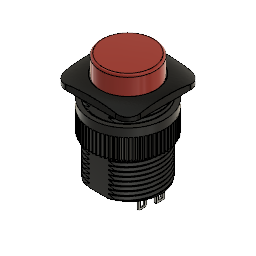
LED Pushbutton (Autodesk Fusion 360 design; units mm, degrees)
Autodesk Fusion 360 part; units mm, degrees
note: some values were not read from the file. Chosen so that the rebuilt part matches the saved one: which face or edge a step refers to. Set by a fixed rule: which sketch regions a step uses.
sketch "Sketch1" plane through (0, 0, 0) normal (0, 0, 1) x (1, 0, 0) in component "Top"
  circle A0 centre (0, 0) radius 6.5
  dimension "d1" = 13
  constraint coincident A0.centre origin
  measures "d1" diameter of A0
extrude "Extrude1" add sketch "Sketch1" along normal blind 6.3 makes body 1 in component "Top"
sketch "Sketch1 (2)" plane through (0, 0, 0) normal (0, 0, 1) x (1, 0, 0) in component "Bezel"
  line L0 (9, 9) -> (-9, 9)
  line L1 (-9, 9) -> (-9, -9)
  line L2 (-9, -9) -> (9, -9)
  line L3 (9, -9) -> (9, 9)
  line L4 (9, 9) -> (-9, -9) construction
  line L5 (-9, 9) -> (9, -9) construction
  dimension "d4" = 18
  dimension "d5" = 18
  constraint horizontal L0
  constraint perpendicular L0 L1
  constraint parallel L0 L2
  constraint parallel L1 L3
  constraint coincident L4 origin
  constraint coincident L5 origin
  measures "d4" distance of L0 L2
  measures "d5" distance of L1 L3
extrude "Extrude1'" add sketch "Sketch1 (2)" along normal blind 1 separate body makes body 2 in component "Bezel"
extrude "Extrude2" add 1 faces at (-3, 3, 1) along direction (0, 0, 1) blind 1 separate body on bodies 2 makes body 3 in component "Bezel"
fillet "Fillet1" radius 3 8 edges at (-9, 9, 0.5) (9, 9, 0.5) (9, -9, 0.5) (-9, -9, 0.5) (-9, 9, 1.5) (9, 9, 1.5) (9, -9, 1.5) (-9, -9, 1.5) on bodies 2 3 in component "Bezel"
combine "Combine1" operation cut target body 3 tool bodies 1 keep tools in component "Bezel"
combine "Combine2" operation cut target body 2 tool bodies 1 keep tools in component "Bezel"
ref_plane "WorkPlane1" through (0, 0, 1) normal (0.707107, -0.707107, 0) x (0.707107, 0.707107, 0) in component "Bezel"
sketch "Sketch2" plane through (0, 0, 1) normal (0.707107, -0.707107, 0) x (0.707107, 0.707107, 0) in component "Bezel"
  line L0 (-10.6066, 1) -> (-10.6066, 0)
  line L1 (-10.6066, 0) -> (-2.1213, 0)
  line L2 (-2.1213, 0) -> (-2.1213, 1)
  line L3 (-2.1213, 1) -> (-10.6066, 1)
  line L4 (-11.4853, 1) -> (-10.6066, 1)
  line L5 (-10.6066, 1) -> (-10.6066, 0)
  line L6 (-10.6066, 0) -> (-11.4853, 0)
  line L7 (-10.6066, 0) -> (-10.6066, 1)
  line L8 (-2.1213, 1) -> (2.1213, 1)
  line L9 (-2.1213, 1) -> (-2.1213, 0)
  line L10 (2.1213, 0) -> (-2.1213, 0)
  line L11 (2.1213, 0) -> (2.1213, 1)
  line L12 (2.1213, 1) -> (2.1213, 0)
  line L13 (2.1213, 0) -> (10.6066, 0)
  line L14 (10.6066, 0) -> (10.6066, 1)
  line L15 (10.6066, 1) -> (2.1213, 1)
  line L16 (10.6066, 1) -> (11.4853, 1)
  line L17 (10.6066, 1) -> (10.6066, 0)
  line L18 (11.4853, 0) -> (10.6066, 0)
  line L19 (10.6066, 0) -> (10.6066, 1)
  arc A0 (-6.364, 1) -> (-11.4853, 0) centre (-6.364, -12.614) ccw
  line L20 (-11.4853, 0) -> (-11.4853, 1)
  line L21 (-11.4853, 1) -> (-6.364, 1)
  constraint tangent L3 A0
  constraint coincident L6.end A0.end
  constraint midpoint L3 A0.start
  constraint coincident L4.start L20.end
revolve "Revolve1" cut sketch "Sketch2" angle 360 about axis through (0, 0, 1.75) along (0, 0, 1) contours L0 L3 L5 L7 A0 L21 | L0 L4 L5 L7 A0 L20 L21 bodies 3 in component "Bezel"
fillet "Fillet1'" radius 0.5 1 edges at (-6.0601, -2.3505, 6.3) on bodies 1 in component "Top"
sketch "Sketch1 (3)" plane through (0, 0, 0) normal (0, 0, 1) x (1, 0, 0) in component "Barrel"
  circle A0 centre (0, 0) radius 7.95
  dimension "d15" = 15.9
  constraint coincident A0.centre origin
  measures "d15" diameter of A0
extrude "Extrude1''" add sketch "Sketch1 (3)" against normal blind 19.5 separate body makes body 4 in component "Barrel"
thread "Thread2" "ANSI Metric M Profile 16.0 M16x1 6g" major diameter 15.884 minor diameter 14.741 pitch 1 angle 60 modelled right hand crest width 0.1429 on face at (7.9401, -0.3963, -13) crest through (7.942, 0, -19.75) on bodies 4 in component "Barrel"
ref_plane "WorkPlane1" through (0, 0, -3) normal (0, 0, 1) x (1, 0, 0)
sketch "Sketch1 (4)" plane through (0, 0, -3) normal (0, 0, 1) x (1, 0, 0) in component "Lock Nut"
  circle A0 centre (0, 0) radius 9
  dimension "d20" = 18
  constraint coincident A0.centre origin
  measures "d20" diameter of A0
extrude "Extrude1'''" add sketch "Sketch1 (4)" against normal blind 2 separate body makes body 5 in component "Lock Nut"
extrude "Extrude2'" add 1 faces at (-5.1676, 0.3267, -5) along direction (0, 0, -1) blind 5 separate body on bodies 5 makes body 6 in component "Lock Nut"
sketch "Sketch2 (2)" plane through (0, 0, -10) normal (0, 0, -1) x (1, 0, 0) in component "Lock Nut"
  line L0 (-0.3464, 9.0821) -> (0, 8.4821)
  line L1 (0, 8.4821) -> (0.3464, 9.0821)
  line L2 (0.3464, 9.0821) -> (-0.3464, 9.0821)
  line L3 (0, 12.5315) -> (0, 0) construction
  dimension "d25" = 60
  dimension "d26" = 60
  dimension "d27" = 0.6
  constraint horizontal L2
  constraint vertical L3
  constraint coincident L3.end origin
  constraint coincident L0.end L3
  measures "d25" angle of L0 L1
  measures "d26" angle of L1 L2
  measures "d27" distance of L0.end L2
extrude "Extrude3" cut sketch "Sketch2 (2)" against normal through all bodies 6 in component "Lock Nut"
pattern_circular "C-Pattern1" count 67 over 360 about axis through (0, 0, 1.75) along (0, 0, 1) of "Extrude3" in component "Lock Nut"
combine "Combine1'" operation add target body 5 tool bodies 6 in component "Lock Nut"
combine "Combine2'" operation cut target body 5 tool bodies 4 keep tools in component "Lock Nut"
combine "Combine3" operation add target body 2 tool bodies 3 in component "Bezel"
sketch "Sketch1 (5)" plane through (0, 0, -19.5) normal (0, 0, -1) x (1, 0, 0) in component "Lug"
  line L0 (-3, 0.5) -> (-2.7, 0.5)
  line L1 (-2.7, 0.5) -> (-2.7, -1.5)
  line L2 (-2.7, -1.5) -> (-3, -1.5)
  line L3 (-3, -1.5) -> (-3, 0.5)
  line L4 (-3.6, -3.25) -> (-3, -3.25)
  line L5 (-3, -3.25) -> (-3, -5.25)
  line L6 (-3, -5.25) -> (-3.6, -5.25)
  line L7 (-3.6, -5.25) -> (-3.6, -3.25)
  dimension "d31" = 0.3
  dimension "d32" = 2
  dimension "d34" = 0.5
  dimension "d35" = 0.6
  dimension "d36" = 3
  dimension "d37" = 2
  dimension "d38" = 3
  dimension "d39" = 1.75
  constraint horizontal L0
  constraint vertical L1
  constraint horizontal L2
  constraint vertical L3
  constraint horizontal L4
  constraint vertical L5
  constraint horizontal L6
  constraint vertical L7
  measures "d31" distance of L0.start L0.end
  measures "d32" distance of L0.start L2.end
  measures "d34" distance of origin L0
  measures "d35" distance of L4.start L4.end
  measures "d36" distance of origin L3
  measures "d37" distance of L4.start L6.end
  measures "d38" distance of origin L5
  measures "d39" distance of L2 L4
extrude "Extrude1''''" add sketch "Sketch1 (5)" along normal blind 5.5 separate body contours L4 L5 L6 L7 makes body 7 in component "Lug"
sketch "Sketch2 (3)" plane through (-3, 0, 0) normal (1, 0, 0) x (0, 1, 0) in component "Lug"
  line L0 (3.75, -22.5) -> (4.75, -22.5)
  line L1 (4.75, -22.5) -> (4.75, -24.5)
  line L2 (4.75, -24.5) -> (3.75, -24.5)
  line L3 (3.75, -24.5) -> (3.75, -22.5)
  line L4 (5.25, -19.5) -> (3.25, -19.5)
  line L5 (3.25, -19.5) -> (3.25, -25)
  line L6 (3.25, -25) -> (5.25, -25)
  line L7 (5.25, -25) -> (5.25, -19.5)
  arc A0 (3.25, -24.9987) -> (5.25, -23.9209) centre (3.327, -22.747) ccw
  line L8 (5.25, -23.9209) -> (5.25, -25)
  line L9 (3.25, -25) -> (3.25, -24.9987)
  dimension "d42" = 1
  dimension "d43" = 2
  dimension "d44" = 0.5
  dimension "d45" = 0.5
  constraint horizontal L0
  constraint vertical L1
  constraint horizontal L2
  constraint vertical L3
  constraint tangent L6 A0
  constraint coincident L7 A0.end
  constraint coincident L5 A0.start
  constraint coincident L6.end L7.start
  constraint coincident L5.end L6.start
  measures "d42" distance of L0.start L0.end
  measures "d43" distance of L0.end L1.end
  measures "d44" distance of L1 L7
  measures "d45" distance of L2 L6
extrude "Extrude2''" cut sketch "Sketch2 (3)" against normal through all contours L0 L1 L2 L3 A0 | L1 L2 A0 bodies 7 in component "Lug"
mirror "MirrorComponent1" about plane through (0, 0, 0) normal (0, 0, 1) of bodies 7 makes body 8 in component "Lug(Mirror)"
extrude "Extrude1'''''" add sketch "Sketch1 (5)" along normal blind 5.5 separate body contours L0 L1 L2 L3 makes body 9 in component "Lug 2"
sketch "Sketch1 (6)" plane through (-2.7, 0, 0) normal (1, 0, 0) x (0, 1, 0) in component "Lug 2"
  line L0 (1.5, -19.5) -> (-0.5, -19.5)
  line L1 (-0.5, -19.5) -> (-0.5, -25)
  line L2 (-0.5, -25) -> (1.5, -25)
  line L3 (1.5, -25) -> (1.5, -19.5)
  line L4 (0, -22.5) -> (1, -22.5)
  line L5 (1, -22.5) -> (1, -24.5)
  line L6 (1, -24.5) -> (0, -24.5)
  line L7 (0, -24.5) -> (0, -22.5)
  arc A0 (-0.5, -24.75) -> (1.5, -24.75) centre (0.5, -22.875) ccw
  dimension "d50" = 0.5
  dimension "d51" = 0.5
  dimension "d52" = 2
  dimension "d53" = 1
  dimension "d55" = 0.25
  dimension "d56" = 0.25
  constraint horizontal L4
  constraint vertical L5
  constraint horizontal L6
  constraint vertical L7
  constraint tangent L2 A0
  constraint coincident L3 A0.end
  constraint coincident L1 A0.start
  measures "d50" distance of L2 L6
  measures "d51" distance of L3 L5
  measures "d52" distance of L4.start L6.end
  measures "d53" distance of L5.end L6.end
  measures "d55" distance of L1.end A0.start
  measures "d56" distance of L2.end A0.end
extrude "Extrude2'''" cut sketch "Sketch1 (6)" against normal through all contours L4 L5 L6 L7 bodies 9 in component "Lug 2"
extrude "Extrude3'" cut sketch "Sketch1 (6)" against normal through all contours L2 L3 A0 | L1 L2 A0 bodies 9 in component "Lug 2"
mirror "MirrorComponent2" about plane through (0, 0, 0) normal (0, 0, 1) of bodies 9 makes body 10 in component "Lug 2(Mirror)"
sketch "Sketch2 (4)" plane through (0, 0, 0) normal (0, 0, 1) x (-1, 0, 0) in component "Barrel"
  line L0 (10.7744, -11.1102) -> (-9.9763, -11.1102)
  line L1 (-9.9763, -11.1102) -> (-9.9763, -7)
  line L2 (-9.9763, -7) -> (10.7744, -7)
  line L3 (10.7744, -7) -> (10.7744, -11.1102)
  line L4 (10.1758, 7) -> (-9.9763, 7)
  line L5 (-9.9763, 7) -> (-9.9763, 10.1126)
  line L6 (-9.9763, 10.1126) -> (10.1758, 10.1126)
  line L7 (10.1758, 10.1126) -> (10.1758, 7)
  dimension "d58" = 7
  dimension "d59" = 7
  constraint horizontal L0
  constraint vertical L1
  constraint horizontal L2
  constraint vertical L3
  constraint horizontal L4
  constraint vertical L5
  constraint horizontal L6
  constraint vertical L7
  measures "d58" distance of origin L2
  measures "d59" distance of origin L4
extrude "Extrude2''''" cut sketch "Sketch2 (4)" against normal through all bodies 4 in component "Barrel"
fillet "Fillet2" radius 0.25 1 edges at (-6.0601, -2.3505, 1.9993) on bodies 2 in component "Bezel"
component "Top" placed x (1, 0, 0) y (0, 1, 0) z (0, 0, 1) at (0, 0, 0)
component "Bezel" placed x (1, 0, 0) y (0, 1, 0) z (0, 0, 1) at (0, 0, 0)
component "Barrel" placed x (1, 0, 0) y (0, 1, 0) z (0, 0, 1) at (0, 0, 0)
component "Lock Nut" placed x (1, 0, 0) y (0, 1, 0) z (0, 0, 1) at (0, 0, 0)
component "Lug" placed x (1, 0, 0) y (0, 1, 0) z (0, 0, 1) at (0, 0, 0)
component "Lug 2" placed x (1, 0, 0) y (0, 1, 0) z (0, 0, 1) at (0, 0, 0)
component "Lug(Mirror)" placed x (-1, 0, 0) y (0, 1, 0) z (0, 0, -1) at (0, 0, 0)
component "Lug 2(Mirror)" placed x (-1, 0, 0) y (0, 1, 0) z (0, 0, -1) at (0, 0, 0)
equation "d5 = d4"
